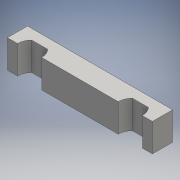
# Autodesk Inventor part: motorHolderTest1
Saved by Autodesk Inventor 2016 (Build 200138000, 138)
## iProperties
Created: 2016-04-11
Part Number: motorHolderTest1
Material: Generic
Document SubType Name: Modeling
Designer: hesaon
Density: 1 g/cm^3
Appearance: Default
Author: hesaon
Autodesk Inventor part; units mm, degrees
ref_plane "YZ Plane" through (0, 0, 0) normal (1, 0, 0) x (0, 1, 0)
ref_plane "XZ Plane" through (0, 0, 0) normal (0, 1, 0) x (-1, 0, 0)
ref_plane "XY Plane" through (0, 0, 0) normal (0, 0, 1) x (1, 0, 0)
sketch "Sketch1" plane through (0, 0, 0) normal (0, 0, 1) x (1, 0, 0)
  line L0 (10, 5) -> (2, 5)
  arc A0 (2, 5) -> (0, 0) centre (7.25, 0) ccw
  arc A1 (12, 0) -> (10, 5) centre (4.75, 0) ccw
  line L1 (0, 0) -> (-5, 0)
  line L2 (-5, 0) -> (-5, 10)
  line L3 (-5, 10) -> (17, 10)
  line L4 (17, 10) -> (17, 0)
  line L5 (17, 0) -> (12, 0)
  dimension "d5" = 5
  dimension "d6" = 10
  dimension "d7" = 22
  dimension "d8" = 2
  dimension "d9" = 2
  dimension "d10" = 8
  dimension "d11" = 5
  dimension "d12" = 7.25
  dimension "d13" = 7.25
  constraints: 12 end point, 4 perpendicular, 4 point on circle, 2 centre point, 1 horizontal, 1 parallel, 1 point on line
  measures "d5" distance of L1.start L1.end
  measures "d6" distance of L1.end L2.end
  measures "d7" distance of L2.end L3.end
  measures "d8" horizontal distance of L1.start L0.end
  measures "d9" horizontal distance of L5.end L0.start
  measures "d10" distance of L0.start L0.end
  measures "d11" vertical distance of L1.start L0.end
  measures "d12" radius of A0
  measures "d13" radius of A1
extrude "Extrusion1" add sketch "Sketch1" along normal blind 14
sketch "Sketch2" plane through (17, 0, 0) normal (1, 0, 0) x (0, 0, -1)
  line L0 (-14, 10) -> (-14, 0) projected
  line L1 (-14, 0) -> (0, 0)
  line L2 (0, 0) -> (0, 10)
  line L3 (0, 10) -> (-14, 10)
  line L4 (-14, 10) -> (-14, 0)
  dimension "d16" = 10
  dimension "d17" = 14
  constraints: 8 end point, 2 parallel, 1 horizontal, 1 perpendicular
  measures "d16" distance of L2.end point (0, 0)
  measures "d17" distance of L2.end L0.start
extrude "Extrusion2" add sketch "Sketch2" along normal blind 50
sketch "Sketch5" plane through (0, 0, 14) normal (0, 0, 1) x (1, 0, 0)
  line L0 (62, 0) -> (67, 0)
  line L1 (12, 0) -> (67, 0) projected
  arc A0 (12, 0) -> (10, 5) centre (4.75, 0) ccw projected
  arc A1 (2, 5) -> (0, 0) centre (7.25, 0) ccw projected
  line L2 (2, 5) -> (10, 5) projected
  arc A2 (62, 0) -> (60, 5) centre (54.75, 0) ccw
  arc A3 (52, 5) -> (50, 0) centre (57.25, 0) ccw
  line L3 (52, 5) -> (60, 5)
  line L4 (50, 0) -> (62, 0)
  dimension "d31" = 0
  dimension "d32" = 0
  dimension "d33" = 5
  dimension "d34" = 50
  dimension "d35" = 0
  dimension "d36" = 0
  dimension "d38" = 7.25
  dimension "d39" = 7.25
  dimension "d40" = 8
  dimension "d41" = 38
  dimension "d42" = 5
  dimension "d43" = 5
  dimension "d44" = 2
  dimension "d45" = 2
  constraints: 6 end point, 4 point on circle, 2 centre point
  measures "d31" distance from line of L1 L0.end
  measures "d32" distance of L1.end L0.end
  measures "d33" distance of L0.end L0.start
  measures "d34" distance of L0.start L1.start
  measures "d35" distance of L0.start L4.end
  measures "d36" distance of L0.start L4.end
  measures "d38" radius of A2
  measures "d39" radius of A3
  measures "d40" distance of L3.start L3.end
  measures "d41" distance of L1.start L4.start
  measures "d42" vertical distance of L4.start L3.start
  measures "d43" vertical distance of L0.start L3.end
  measures "d44" horizontal distance of L4.start L3.start
  measures "d45" horizontal distance of L0.start L3.end
extrude "Extrusion3" cut sketch "Sketch5" against normal through all
body "Solid1"
